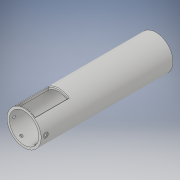
# Autodesk Inventor part: reservoir_guide
Saved by Autodesk Inventor 2019 (Build 230136000, 136)
## iProperties
Created: 2019-03-19
Part Number: reservoir_guide
Material: Générique
Document SubType Name: Modeling
Designer: theor
Density: 1 g/cm^3
Appearance: Par défaut
Author: theor
Autodesk Inventor part; units mm, degrees
ref_plane "XY Plane" through (0, 0, 0) normal (0, 0, 1) x (1, 0, 0)
sketch "Esquisse1" plane through (0, 0, 0) normal (1, 0, 0) x (0, 1, 0)
  line L0 (0, 0) -> (0, 594.5025)
  line L1 (22, 0) -> (22, 170)
  line L2 (19, 0) -> (19, 170)
  line L3 (22, 170) -> (19, 170)
  line L4 (22, 0) -> (19, 0)
  dimension "d0" = 38
  dimension "d3" = 3
  dimension "d58" = 170
  constraints: 10 end point, 3 vertical, 2 horizontal, 1 horizontal alignment
  measures "d0" diameter of L2 L0
  measures "d3" distance between parallel lines of L1 L2
  measures "d58" distance of L2.start L2.end
revolve "Révolution1" add sketch "Esquisse1" angle 360 about axis through (0, 0, 0) along (0, 0, 1)
sketch "Esquisse3" plane through (0, 0, 0) normal (0, 1, 0) x (-1, 0, 0)
  line L0 (-19, 170) -> (19, 170) projected
  line L1 (12.5, 168) -> (-12.5, 168)
  line L2 (-12.5, 168) -> (-12.5, 126)
  line L3 (-12.5, 126) -> (12.5, 126)
  line L4 (12.5, 126) -> (12.5, 168)
  point P0 (0, 0)
  point P1 (0, 168)
  point P2 (0, 170)
  dimension "d108" = 42
  dimension "d109" = 2
  dimension "d110" = 25
  constraints: 8 end point, 2 midpoint, 2 parallel, 1 horizontal, 1 perpendicular, 1 vertical alignment
  measures "d108" distance of L3.end L1.start
  measures "d109" distance between parallel lines of L0 L1
  measures "d110" distance of L2.end L3.end
extrude "Extrusion2" cut sketch "Esquisse3" along normal up to surface
ref_plane "Plan de construction2" through (22, 0, 85) normal (1, 0, 0) x (0, 1, 0)
sketch "Esquisse4" plane through (22, 0, 85) normal (1, 0, 0) x (0, 1, 0)
  line L0 (-22, 85) -> (22, 85) projected
  point P0 (0, -85)
  point P1 (0, 79)
  dimension "d24" = 6
  constraints: 1 vertical alignment
  measures "d24" distance from line of L0 point (0, 79)
hole "Perçage1" at (22, 0, 164) direction (-1, 0, 0) diameter 3.4 depth 8 counterbore diameter 6.5 counterbore depth 0.5 clearance for "Vis d'assemblage à six pans creux ISO 4762" size "M3" standard "ISO"
pattern_circular "Réseau circulaire2" count 4 over 180 about axis through (0, 0, -10) along (0, 0, -1) of "Perçage1"
chamfer "Chanfrein2" distance 1 angle 45 6 edges at (-12.5, 18.1039, 147) (-6.5466, 21.0034, 126) (6.5466, 21.0034, 126) (12.5, 18.1039, 147) (-6.5466, 21.0034, 168) (6.5466, 21.0034, 168)
ref_plane "Plan de construction3" through (0, -22, 85) normal (0, 1, 0) x (-1, 0, 0)
thread "Filetage3" size "M38x1.5" class "6H" standard "ISO Metric profile" length 10
